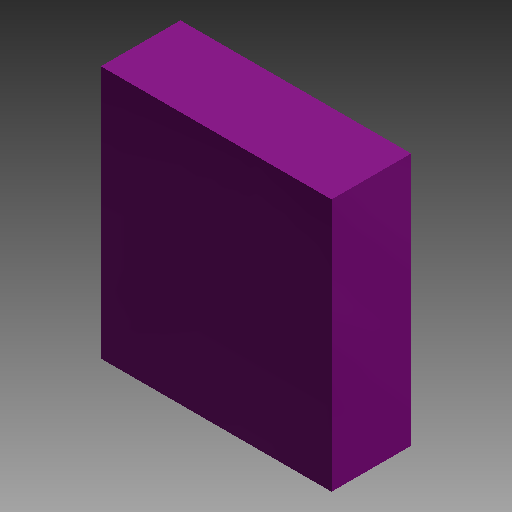
# Autodesk Inventor part: LM25011MY/NOPB
Saved by Autodesk Inventor 2018.2 (Build 222227000, 227)
## iProperties
Part Number: LM25011MY/NOPB
Material: Generic
Document SubType Name: Modeling
Designer: autocad
Appearance: VSSOP10, LM25011MY_NOPB
Author: autocad
Autodesk Inventor part; units mm, degrees
ref_plane "YZ Plane" through (0, 0, 0) normal (1, 0, 0) x (0, 1, 0)
ref_plane "XZ Plane" through (0, 0, 0) normal (0, 1, 0) x (-1, 0, 0)
ref_plane "XY Plane" through (0, 0, 0) normal (0, 0, 1) x (1, 0, 0)
sketch "VSSOP10, LM25011MY_NOPB_51" plane through (0, 0, 0) normal (0, 0, 1) x (1, 0, 0)
  line L0 (-1.55, 1.7) -> (1.55, 1.7)
  line L1 (1.55, 1.7) -> (1.55, -1.7)
  line L2 (1.55, -1.7) -> (-1.55, -1.7)
  line L3 (-1.55, -1.7) -> (-1.55, 1.7)
  constraints: 8 end point
extrude "Extrusion1" add sketch "VSSOP10, LM25011MY_NOPB_51" along normal blind 1.07
body "Solid1"
